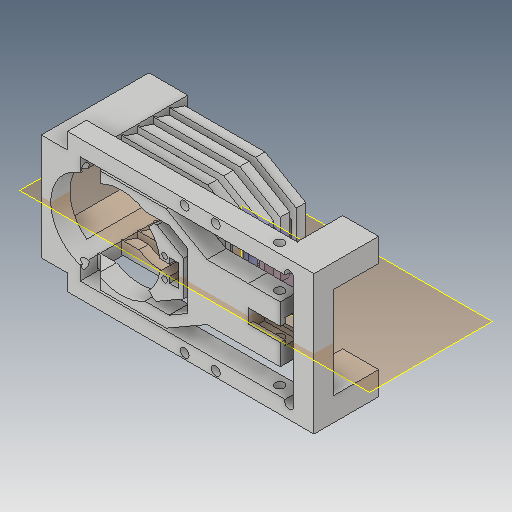
# Autodesk Inventor part: 20_focus_inlet_linearflexure_v1_1x1
Saved by Autodesk Inventor 2019.4 (Build 234330000, 330)
## iProperties
Created: 2020-02-03
Part Number: 20_focus_inlet_linearflexure_v1_1x1
Material: Generic
Document SubType Name: Modeling
Designer: diederichbenedict
Density: 1 g/cm^3
Appearance: Default
Author: diederichbenedict
Autodesk Inventor part; units mm, degrees
ref_plane "Work Plane1" through (0, 0, 0) normal (0, 0, 1) x (1, 0, 0)
sketch "Sketch1" plane through (0, 0, 0) normal (0, 0, 1) x (1, 0, 0)
  line L0 (33.5, -15.3849) -> (35.5, -15.3849) projected
  line L1 (35.5, -15.3849) -> (35.5, -14.1603) projected
  arc A0 (35.5, -14.1603) -> (35.3294, -13.8326) centre (35.1, -14.1603) ccw projected
  line L2 (35.3294, -13.8326) -> (34.0923, -12.9664) projected
  arc A1 (33.8775, -12.693) -> (34.0923, -12.9664) centre (34.4364, -12.4749) ccw projected
  arc A2 (33.8775, -12.693) -> (33.8775, -21.107) centre (23.1, -16.9) ccw projected
  arc A3 (34.0923, -20.8336) -> (33.8775, -21.107) centre (34.4364, -21.3251) ccw construction
  line L3 (34.0923, -20.8336) -> (35.3294, -19.9674) construction
  arc A4 (35.3294, -19.9674) -> (35.5, -19.6397) centre (35.1, -19.6397) ccw construction
  line L4 (35.5, -19.6397) -> (35.5, -18.4151) construction
  line L5 (35.5, -18.4151) -> (33.5, -18.4151) construction
  line L6 (33.5, -18.4151) -> (33.5, -15.3849) projected
  line L7 (30.0099, -20.9316) -> (30.0099, -25.4) construction
  line L8 (30.0099, -25.4) -> (27.6057, -25.4) construction
  line L9 (27.6057, -25.4) -> (27.6057, -23.5105) construction
  arc A5 (27.6057, -10.2895) -> (27.6057, -23.5105) centre (23.1, -16.9) ccw construction
  line L10 (27.6057, -10.2895) -> (27.6057, -8.4) construction
  line L11 (27.6057, -8.4) -> (30.0099, -8.4) construction
  line L12 (30.0099, -8.4) -> (30.0099, -12.8684) projected
  arc A6 (30.0099, -20.9316) -> (30.0099, -12.8684) centre (23.1, -16.9) ccw projected
  line L13 (23.1, -16.9) -> (97.1528, -16.9) construction
  line L14 (35.4811, -18.415) -> (35.4811, -19.6397) construction
  arc A7 (35.3186, -19.9519) -> (35.4811, -19.6397) centre (35.1, -19.6397) ccw construction
  line L15 (35.3186, -19.9519) -> (34.0815, -20.8182) construction
  arc A8 (34.0815, -20.8182) -> (33.8599, -21.1001) centre (34.4364, -21.3251) ccw construction
  line L16 (35.7169, -15.385) -> (35.7169, -16.9) construction
  line L17 (35.7169, -15.385) -> (35.7169, -16.9)
  line L18 (23.1, -16.9) -> (31.3304, -8.6696)
  line L19 (23.1, -16.9) -> (34.7396, -16.9) construction
  line L20 (31.3304, -8.6696) -> (33.4518, -6.5482)
  line L21 (33.4518, -6.5482) -> (34.3134, -6.5482)
  line L22 (42.7169, -11.4) -> (42.7169, -16.9)
  line L23 (35.7169, -16.9) -> (42.7169, -16.9)
  line L24 (35.7169, -16.9) -> (41.2169, -16.9)
  line L25 (41.2169, -16.9) -> (41.2169, -15.2)
  line L26 (41.2169, -15.2) -> (35.7169, -15.2)
  line L27 (35.7169, -15.2) -> (35.7169, -16.9)
  line L28 (41.2169, -15.2) -> (38.2169, -15.2)
  line L29 (38.2169, -15.2) -> (38.2169, -13.4)
  line L30 (38.2169, -13.4) -> (41.2169, -13.4)
  line L31 (41.2169, -13.4) -> (41.2169, -15.2)
  line L32 (33.4518, -6.5482) -> (34.3134, -6.5482) construction
  line L33 (42.7169, -11.4) -> (34.3134, -6.5482)
  line L34 (42.7169, -11.4) -> (52.4204, -11.4) construction
  arc A9 (31.3304, -8.6696) -> (30.0099, -7.5334) centre (23.1, -16.9) ccw construction
  arc A10 (28.2242, -6.5482) -> (33.8599, -21.1001) centre (23.1, -16.9) ccw construction
  arc A11 (33.8599, -21.1001) -> (33.9142, -20.9583) centre (23.1, -16.9) ccw
  arc A12 (34.6422, -15.3971) -> (31.3304, -8.6696) centre (23.1, -16.9) ccw
  line L35 (35.7169, -15.2) -> (34.6148, -15.2)
  circle A13 centre (36.7119, -13.6943) radius 0.9
  point P0 (0, 0)
  dimension "d1" = 45
  dimension "d2" = 3
  dimension "d6" = 1.7
  dimension "d8" = 3.5
  dimension "d9" = 3
  dimension "d147" = 7
  dimension "d148" = 120
  dimension "d149" = 5.5
  dimension "d155" = 12.6169
  dimension "d156" = 1.8
  dimension "d162" = 1.5
  constraints: 46 end point, 13 point on circle, 8 horizontal, 7 centre point, 6 point on line, 4 parallel, 4 perpendicular, 2 collinear, 2 equal length, 1 coincident, 3 other
  measures "d1" angle of L19 L18
  measures "d2" distance of L18.end L20.end
  measures "d6" distance of L25.end L24.end
  measures "d8" distance between parallel lines of L13 L30
  measures "d9" distance between parallel lines of L31 L29
  measures "d147" distance of L16.end L22.end
  measures "d148" angle of L22 L33
  measures "d149" distance of L22.start L22.end
  measures "d155" distance from line of L16 A2.centre
  measures "d156" diameter of A13
  measures "d162" distance between parallel lines of L31 L22
extrude "Extrusion1" add sketch "Sketch1" against normal blind 35 contours A12 A1 L2 A0 L1 L35 | L1 A0 L2 A1 A12 L20 L21 L33 L22 L23 L25 L31 L30 L29 L26 L35
sketch "Sketch2" plane through (0, 0, 0) normal (0, 0, 1) x (1, 0, 0)
  line L0 (41.2169, -13.4) -> (41.2169, -16.9) projected
  line L1 (42.7169, -16.9) -> (41.2169, -16.9) projected
  line L2 (42.7169, -11.4) -> (42.7169, -16.9) projected
  line L3 (31.3304, -8.6696) -> (33.4518, -6.5482) projected
  line L4 (34.6148, -15.2) -> (38.2169, -15.2) projected
  line L5 (38.2169, -15.2) -> (38.2169, -13.4) projected
  line L6 (38.2169, -13.4) -> (41.2169, -13.4) projected
  line L7 (95.8, 0) -> (0, 0) projected
  line L8 (6, -33.8) -> (89.8, -33.8) projected
  line L9 (6, -33.8) -> (6, 0) projected
  line L10 (11, -0.7) -> (45.4618, -0.7)
  line L11 (11, -4.7) -> (11, -0.7)
  line L12 (44.0169, -4.6174) -> (44.0169, -16.9)
  line L13 (44.0169, -16.9) -> (50.0084, -16.9)
  line L14 (50.0084, -16.9) -> (50.0084, -8.0766)
  line L15 (6.2, -0.1) -> (10.2, -0.1)
  line L16 (10.2, -0.1) -> (10.2, -16.9)
  line L17 (10.2, -16.9) -> (6.2, -16.9)
  line L18 (6.2, -16.9) -> (6.2, -0.1)
  line L19 (50.0084, -16.9) -> (63.0169, -16.9)
  line L20 (63.0169, -16.9) -> (63.0169, -8.0766)
  line L21 (63.0169, -8.0766) -> (50.0084, -8.0766)
  line L22 (50.0084, -8.0766) -> (50.0084, -16.9)
  arc A0 (79.6921, -19.4) -> (79.6921, -14.4) centre (79.6921, -16.9) ccw projected
  line L23 (58.0169, -7.7662) -> (58.0169, -8.0766)
  line L24 (6.2, -0.1) -> (10.2, -0.1)
  line L25 (10.2, -0.1) -> (10.2, 4.9)
  line L26 (10.2, 4.9) -> (6.2, 4.9)
  line L27 (6.2, 4.9) -> (6.2, -0.1)
  line L28 (1.6162, -33.8) -> (1.6162, 0) projected
  line L29 (-2, 0) -> (1.6162, 0) projected
  line L30 (-2, -33.8) -> (-2, 0) projected
  line L31 (1.6162, -33.8) -> (-2, -33.8) projected
  line L32 (6.2, -16.9) -> (-2, -16.9)
  line L33 (-2, -16.9) -> (-2, -0.2)
  line L34 (-2, -0.2) -> (6.2, -0.2)
  line L35 (6.2, -0.2) -> (6.2, -16.9)
  line L36 (-2, 0) -> (0, 0) projected
  line L37 (10.2, 4.9) -> (89.6, 4.9)
  line L38 (89.6, 4.9) -> (89.6, 0)
  line L39 (89.6, 0) -> (10.2, 0)
  line L40 (10.2, 0) -> (10.2, 4.9)
  line L41 (89.8, 0) -> (89.8, 4.5) projected
  line L42 (95.8, 0) -> (89.8, 0) projected
  line L43 (97.8, -41.8) -> (97.8, 0) construction
  line L44 (94.1838, 0) -> (94.1838, -33.8) projected
  line L45 (97.8, -33.8) -> (94.1838, -33.8) projected
  line L46 (97.8, -33.8) -> (97.8, 0) projected
  line L47 (94.1838, 0) -> (97.8, 0) projected
  line L48 (97.8, -0.2) -> (85.8, -0.2)
  line L49 (85.8, -0.2) -> (85.8, -4.2)
  line L50 (85.8, -4.2) -> (97.8, -4.2)
  line L51 (97.8, -4.2) -> (97.8, -0.2)
  line L52 (85.8, -0.2) -> (89.6, -0.2)
  line L53 (89.6, -0.2) -> (89.6, 0)
  line L54 (89.6, 0) -> (85.8, 0)
  line L55 (85.8, 0) -> (85.8, -0.2)
  line L56 (34.3134, -6.5482) -> (42.7169, -11.4) projected
  line L57 (33.4518, -6.5482) -> (34.3134, -6.5482) projected
  line L58 (44.0169, -8.0815) -> (38.1599, -4.7)
  line L59 (44.0169, -8.0815) -> (50.78, -8.0815) construction
  line L60 (37.2316, -0.7) -> (50.0084, -8.0766)
  line L61 (37.2316, -0.7) -> (51.9849, -0.7) construction
  line L62 (38.1599, -4.7) -> (11, -4.7)
  line L63 (97.8, -4.2) -> (94.1838, -4.2)
  line L64 (94.1838, -4.2) -> (94.1838, -16.9)
  line L65 (94.1838, -16.9) -> (97.8, -16.9)
  line L66 (97.8, -16.9) -> (97.8, -4.2)
  line L67 (63.0169, -8.0766) -> (58.0169, -8.0766)
  line L68 (58.0169, -8.0766) -> (58.0169, -9.9)
  line L69 (58.0169, -9.9) -> (63.0169, -9.9)
  line L70 (63.0169, -9.9) -> (63.0169, -8.0766)
  circle A1 centre (23.1, -16.9) radius 10 projected
  circle A2 centre (23.1, -16.9) radius 12.5 projected
  arc A3 (30.5513, -4.7) -> (15.6487, -4.7) centre (23.1, -16.9) ccw
  arc A4 (34.6148, -15.2) -> (31.3304, -8.6696) centre (23.1, -16.9) ccw projected
  dimension "d12" = 5
  dimension "d13" = 0.7
  dimension "d15" = 4
  dimension "d16" = 0.2
  dimension "d25" = 5
  dimension "d28" = 0.1
  dimension "d29" = 5
  dimension "d30" = 0.2
  dimension "d31" = 0.2
  dimension "d32" = 12
  dimension "d33" = 4
  dimension "d34" = 0.2
  dimension "d59" = 1.3
  dimension "d68" = 7
  dimension "d150" = 4
  dimension "d151" = 3
  constraints: 94 end point, 22 parallel, 12 horizontal, 11 point on line, 9 perpendicular, 2 equal length, 2 point on circle, 1 centre point, 1 coincident, 1 midpoint
  measures "d12" distance between parallel lines of L11 L9
  measures "d13" distance between parallel lines of L10 L7
  measures "d15" distance of L16.end L17.end
  measures "d16" distance between parallel lines of L18 L9
  measures "d25" distance between parallel lines of L20 L23
  measures "d28" distance between parallel lines of L7 L15
  measures "d29" distance of L25.end L24.end
  measures "d30" distance between parallel lines of L34 L36
  measures "d31" distance between parallel lines of L41 L38
  measures "d32" distance of L50.end L49.end
  measures "d33" distance of L49.end L48.end
  measures "d34" distance between parallel lines of L7 L48
  measures "d59" distance between parallel lines of L12 L2
  measures "d68" distance between parallel lines of L69 L19
  measures "d150" distance between parallel lines of L10 L62
  measures "d151" distance between parallel lines of L60 L58
extrude "Extrusion2" add sketch "Sketch2" against normal blind 6 contours L62 L11 L10 L60 L12 L58 A3 | L12 L60 L14 L13 | L21 L68 L69 L20 L19 L14 | L21 L20 L69 L68 | L48 L46 L50 L44 | L44 L50 L49 L48 | L53 L48 L55 L7 | L7 L25 L37 L38 | L50 L46 L65 L44 | L25 L15 L27 L7 | L7 L27 L26 L25 | L16 L17 L18 L15 | L34 L18 L32 L9 | L9 L32 L28 L34 | L28 L32 L30 L34
sketch "Sketch3" plane through (0, 0, -6) normal (0, 0, 1) x (1, 0, 0)
  line L0 (44.0169, -8.0815) -> (44.0169, -16.9) projected
  line L1 (44.0169, -16.9) -> (63.0169, -16.9) projected
  line L2 (63.0169, -8.0766) -> (63.0169, -16.9) projected
  line L3 (63.0169, -8.0766) -> (50.0084, -8.0766) projected
  line L4 (37.2316, -0.7) -> (11, -0.7) projected
  line L5 (11, -0.7) -> (11, -4.7) projected
  line L6 (41.2169, -13.4) -> (41.2169, -16.9) projected
  line L7 (42.7169, -16.9) -> (41.2169, -16.9) projected
  line L8 (42.7169, -11.4) -> (42.7169, -16.9) projected
  line L9 (31.3304, -8.6696) -> (33.4518, -6.5482) projected
  line L10 (34.6148, -15.2) -> (38.2169, -15.2) projected
  line L11 (38.2169, -15.2) -> (38.2169, -13.4) projected
  line L12 (38.2169, -13.4) -> (41.2169, -13.4) projected
  line L13 (6.2, 4.9) -> (6.2, -0.2) projected
  line L14 (-2, -16.9) -> (10.2, -16.9) projected
  line L15 (10.2, -16.9) -> (10.2, 0) projected
  line L16 (11, -4.7) -> (11, -0.7) projected
  line L17 (10.2, 0) -> (10.2, -16.9) projected
  line L18 (11, -0.7) -> (10.2, -0.7)
  line L19 (10.2, -0.7) -> (10.2, -4.7)
  line L20 (10.2, -4.7) -> (11, -4.7)
  line L21 (11, -4.7) -> (11, -0.7)
  line L22 (44.0169, -16.9) -> (44.0169, -8.0815) projected
  line L23 (42.7169, -16.9) -> (44.0169, -16.9)
  line L24 (44.0169, -16.9) -> (44.0169, -11.4)
  line L25 (44.0169, -11.4) -> (42.7169, -11.4)
  line L26 (42.7169, -11.4) -> (42.7169, -16.9)
  line L27 (6.2, -0.2) -> (-2, -0.2) projected
  line L28 (-2, -0.2) -> (-2, -16.9) projected
  line L29 (89.6, 4.9) -> (6.2, 4.9) projected
  line L30 (10.2, 0) -> (85.8, 0) projected
  line L31 (89.6, -0.2) -> (89.6, 4.9) projected
  line L32 (85.8, 0) -> (85.8, -4.2) projected
  line L33 (85.8, -4.2) -> (94.1838, -4.2) projected
  line L34 (97.8, -16.9) -> (97.8, -0.2) projected
  line L35 (97.8, -0.2) -> (89.6, -0.2) projected
  line L36 (33.4518, -6.5482) -> (34.3134, -6.5482) projected
  line L37 (50.0084, -8.0766) -> (37.2316, -0.7) projected
  line L38 (30.5513, -4.7) -> (38.1599, -4.7) projected
  line L39 (38.1599, -4.7) -> (44.0169, -8.0815) projected
  line L40 (94.1838, -4.2) -> (94.1838, -16.9) projected
  line L41 (94.1838, -16.9) -> (97.8, -16.9) projected
  line L42 (11, -4.7) -> (15.6487, -4.7) projected
  arc A0 (30.5513, -4.7) -> (15.6487, -4.7) centre (23.1, -16.9) ccw projected
  line L43 (34.3134, -6.5482) -> (42.7169, -11.4) projected
  arc A1 (34.6148, -15.2) -> (31.3304, -8.6696) centre (23.1, -16.9) ccw projected
  point P0 (0, 0)
  point P1 (42, -4.4)
  point P2 (10.2, -0.1)
  point P3 (10.2, 4.9)
  dimension "d152" = 0
  constraints: 16 end point, 4 parallel, 2 horizontal, 2 perpendicular, 1 point on line, 2 other
  measures "d152" distance from line of L8.start L25
extrude "Extrusion3" add sketch "Sketch3" along normal blind 0.5 contours L0 L23 L8 L25 | L20 L15 L18 L5
sketch "Sketch5" plane through (0, 0, -6) normal (0, 0, -1) x (-1, 0, 0)
  line L0 (2, -16.9) -> (2, -0.2) projected
  line L1 (2, -0.2) -> (-6.2, -0.2) projected
  line L2 (-6.2, -0.2) -> (-6.2, 4.9) projected
  line L3 (-6.2, 4.9) -> (-89.6, 4.9) projected
  line L4 (-89.6, 4.9) -> (-89.6, -0.2) projected
  line L5 (-89.6, -0.2) -> (-97.8, -0.2) projected
  line L6 (-97.8, -0.2) -> (-97.8, -16.9) projected
  line L7 (-94.1838, -4.2) -> (-85.8, -4.2) projected
  line L8 (-85.8, -4.2) -> (-85.8, 0) projected
  line L9 (-85.8, 0) -> (-10.2, 0) projected
  line L10 (-10.2, 0) -> (-10.2, -0.7) projected
  line L11 (-10.2, -16.9) -> (2, -16.9) projected
  line L12 (-97.8, -16.9) -> (-94.1838, -16.9) projected
  line L13 (-94.1838, -16.9) -> (-94.1838, -4.2) projected
  line L14 (-10.2, -4.7) -> (-10.2, -0.7) projected
  arc A0 (-1, -16.9) -> (-10.2, -4.3971) centre (-14.0958, -16.9) ccw
  line L15 (-10.2, -4.7) -> (-10.2, -16.9) projected
  line L16 (-37.2316, -0.7) -> (-10.2, -0.7) projected
  line L17 (-37.2316, -0.7) -> (-50.0084, -8.0766) projected
  line L18 (-50.0084, -8.0766) -> (-63.0169, -8.0766) projected
  line L19 (-63.0169, -8.0766) -> (-63.0169, -16.9) projected
  line L20 (-63.0169, -16.9) -> (-42.7169, -16.9) projected
  line L21 (-42.7169, -11.4) -> (-42.7169, -16.9) projected
  line L22 (-44.0169, -8.0815) -> (-38.1599, -4.7) projected
  line L23 (-38.1599, -4.7) -> (-30.5513, -4.7) projected
  arc A1 (-15.6487, -4.7) -> (-30.5513, -4.7) centre (-23.1, -16.9) ccw projected
  line L24 (-15.6487, -4.7) -> (-10.2, -4.7) projected
  line L25 (-44.0169, -11.4) -> (-42.7169, -11.4) projected
  line L26 (-44.0169, -11.4) -> (-44.0169, -8.0815) projected
  dimension "d65" = 0
  dimension "d66" = 3
  constraints: 2 point on circle, 1 centre point, 1 point on line
  measures "d65" distance from line of A0.centre L11
  measures "d66" distance from line of L0 A0.start
extrude "Extrusion5" cut sketch "Sketch5" against normal through all contours L11 L15 L14 A0
sketch "Sketch6" plane through (0, 0, -6) normal (0, 0, -1) x (-1, 0, 0)
  line L0 (-50.0084, -8.0766) -> (-63.0169, -8.0766) projected
  line L1 (-63.0169, -8.0766) -> (-63.0169, -16.9) projected
  line L2 (-1, -16.9) -> (2, -16.9) construction
  line L3 (-10.2, 0) -> (-10.2, -0.7) projected
  line L4 (2, -0.2) -> (2, -16.9) projected
  line L5 (2, -0.2) -> (-10.2, -0.2)
  line L6 (2, -4.4) -> (2, -0.2)
  line L7 (2, -4.4) -> (2, -0.2) construction
  line L8 (2, -0.2) -> (-10.2, -0.2) construction
  line L9 (-37.2316, -0.7) -> (-50.0084, -8.0766) projected
  line L10 (-44.0169, -8.0815) -> (-38.1599, -4.7) projected
  line L11 (2, -4.4) -> (-10.2, -4.4)
  line L12 (-10.2, -4.4) -> (-10.2, -0.2)
  line L13 (-10.2, -0.2) -> (2, -0.2)
  line L14 (2, -0.2) -> (2, -4.4)
  line L15 (-38.1599, -4.7) -> (-30.5513, -4.7) projected
  arc A0 (-15.6487, -4.7) -> (-30.5513, -4.7) centre (-23.1, -16.9) ccw projected
  line L16 (-37.2316, -0.7) -> (-10.2, -0.7) projected
  line L17 (-63.0169, -16.9) -> (-42.7169, -16.9) projected
  line L18 (-42.7169, -11.4) -> (-42.7169, -16.9) projected
  line L19 (-15.6487, -4.7) -> (-10.2, -4.7) projected
  line L20 (-1, -16.9) -> (2, -16.9) projected
  line L21 (-37.2316, -0.7) -> (-10.2, -0.7) projected
  line L22 (-37.2316, -0.7) -> (-50.0084, -8.0766) projected
  line L23 (-50.0084, -8.0766) -> (-63.0169, -8.0766) projected
  line L24 (-63.0169, -8.0766) -> (-63.0169, -16.9) projected
  line L25 (-63.0169, -16.9) -> (-42.7169, -16.9) projected
  line L26 (-42.7169, -11.4) -> (-42.7169, -16.9) projected
  line L27 (-44.0169, -8.0815) -> (-38.1599, -4.7) projected
  line L28 (-38.1599, -4.7) -> (-30.5513, -4.7) projected
  arc A1 (-15.6487, -4.7) -> (-30.5513, -4.7) centre (-23.1, -16.9) ccw projected
  line L29 (-15.6487, -4.7) -> (-10.2, -4.7) projected
  line L30 (-10.2, -4.7) -> (-10.2, -4.3971) projected
  arc A2 (-1, -16.9) -> (-10.2, -4.3971) centre (-14.0958, -16.9) ccw projected
  line L31 (-10.2, -4.7) -> (-10.2, -4.3971) projected
  arc A3 (-1, -16.9) -> (-10.2, -4.3971) centre (-14.0958, -16.9) ccw projected
  line L32 (2, -16.9) -> (2, -0.2) projected
  line L33 (2, -0.2) -> (-6.2, -0.2) projected
  line L34 (-6.2, -0.2) -> (-6.2, 4.9) projected
  line L35 (-6.2, 4.9) -> (-89.6, 4.9) projected
  line L36 (-89.6, 4.9) -> (-89.6, -0.2) projected
  line L37 (-89.6, -0.2) -> (-97.8, -0.2) projected
  line L38 (-97.8, -0.2) -> (-97.8, -16.9) projected
  line L39 (-97.8, -16.9) -> (-94.1838, -16.9) projected
  line L40 (-94.1838, -16.9) -> (-94.1838, -4.2) projected
  line L41 (-94.1838, -4.2) -> (-85.8, -4.2) projected
  line L42 (-85.8, -4.2) -> (-85.8, 0) projected
  line L43 (-85.8, 0) -> (-10.2, 0) projected
  line L44 (-10.2, 0) -> (-10.2, -0.7) projected
  line L45 (2, -16.9) -> (2, -0.2) projected
  line L46 (2, -0.2) -> (-6.2, -0.2) projected
  line L47 (-6.2, -0.2) -> (-6.2, 4.9) projected
  line L48 (-6.2, 4.9) -> (-89.6, 4.9) projected
  line L49 (-89.6, 4.9) -> (-89.6, -0.2) projected
  line L50 (-89.6, -0.2) -> (-97.8, -0.2) projected
  line L51 (-97.8, -0.2) -> (-97.8, -16.9) projected
  line L52 (-97.8, -16.9) -> (-94.1838, -16.9) projected
  line L53 (-94.1838, -16.9) -> (-94.1838, -4.2) projected
  line L54 (-94.1838, -4.2) -> (-85.8, -4.2) projected
  line L55 (-85.8, -4.2) -> (-85.8, 0) projected
  line L56 (-85.8, 0) -> (-10.2, 0) projected
  line L57 (-44.0169, -11.4) -> (-42.7169, -11.4) projected
  line L58 (-44.0169, -11.4) -> (-42.7169, -11.4) projected
  line L59 (-44.0169, -11.4) -> (-44.0169, -8.0815) projected
  line L60 (-44.0169, -11.4) -> (-44.0169, -8.0815) projected
  point P0 (0, 0)
  constraints: 16 end point, 2 horizontal, 2 parallel, 1 perpendicular
ref_plane "Work Plane2" through (6, 4.5, -33.8) normal (0, 0, 1) x (1, 0, 0)
extrude "Extrusion6" add sketch "Sketch6" along normal up to surface (27.8 mm away) contours L3 L5 L4 L11 A2 L12 | A2 L11 L12
ref_plane "Work Plane3" through (0, 0, -18) normal (0, 0, -1) x (-1, 0, 0)
sketch "Sketch7" plane through (0, 0, -18) normal (0, 0, -1) x (-1, 0, 0)
  line L0 (-11, -0.7) -> (-10.2, -0.7) projected
  line L1 (-10.2, -4.7) -> (-11, -4.7) projected
  line L2 (-11.9304, -0.7) -> (-11, -0.7) projected
  line L3 (-11.9304, -4.3971) -> (-11.9304, -0.7) projected
  line L4 (-50.0084, -8.0766) -> (-63.0169, -8.0766) projected
  line L5 (-63.0169, -8.0766) -> (-63.0169, -16.9) projected
  line L6 (-42.7169, -16.9) -> (-44.0169, -16.9) projected
  line L7 (-42.7169, -16.9) -> (-42.7169, -11.4) projected
  line L8 (-10.2, -0.2) -> (-10.2, -4.4) projected
  line L9 (2, -4.4) -> (2, -0.2) projected
  line L10 (2, -0.2) -> (-10.2, -0.2) projected
  line L11 (-37.2316, -0.7) -> (-50.0084, -8.0766) projected
  line L12 (-44.0169, -8.0815) -> (-38.1599, -4.7) projected
  line L13 (-11, -4.3971) -> (-11.9304, -4.3971) projected
  line L14 (-10.2, -4.4) -> (2, -4.4) projected
  line L15 (-38.1599, -4.7) -> (-30.5513, -4.7) projected
  arc A0 (-15.6487, -4.7) -> (-30.5513, -4.7) centre (-23.1, -16.9) ccw projected
  line L16 (-11, -0.7) -> (-11, -4.3971) projected
  line L17 (-44.0169, -11.4) -> (-44.0169, -16.9) projected
  line L18 (-37.2316, -0.7) -> (-10.2, -0.7) projected
  line L19 (-63.0169, -16.9) -> (-42.7169, -16.9) construction
  line L20 (-42.7169, -11.4) -> (-42.7169, -16.9) projected
  line L21 (-15.6487, -4.7) -> (-10.2, -4.7) projected
  line L22 (-11, -0.7) -> (-11, -4.7) projected
  line L23 (-10.2, -4.3971) -> (-10.2, -0.7) projected
  line L24 (-10.2, -4.4) -> (-10.2, -4.3971) projected
  line L25 (2, -4.4) -> (-10.1907, -4.4) projected
  line L26 (-1, -16.9) -> (2, -16.9) projected
  arc A1 (-1, -16.9) -> (-10.1907, -4.4) centre (-14.0958, -16.9) ccw projected
  line L27 (-10.2, -4.7) -> (-10.2, -4.3971) projected
  line L28 (-10.2, -4.3971) -> (-10.2, -0.7) projected
  line L29 (-10.2, -0.2) -> (-6.2, -0.2) projected
  line L30 (-6.2, -0.2) -> (-6.2, 4.9) projected
  line L31 (-6.2, 4.9) -> (-89.6, 4.9) projected
  line L32 (-89.6, 4.9) -> (-89.6, -0.2) projected
  line L33 (-89.6, -0.2) -> (-97.8, -0.2) projected
  line L34 (-97.8, -0.2) -> (-97.8, -16.9) projected
  line L35 (-97.8, -16.9) -> (-94.1838, -16.9) projected
  line L36 (-94.1838, -16.9) -> (-94.1838, -4.2) projected
  line L37 (-94.1838, -4.2) -> (-85.8, -4.2) projected
  line L38 (-85.8, -4.2) -> (-85.8, 0) projected
  line L39 (-85.8, 0) -> (-10.2, 0) projected
  line L40 (-10.2, 0) -> (-10.2, -0.2) projected
  line L41 (-10.2, -4.7) -> (-10.2, -4.4) projected
  line L42 (2, -16.9) -> (2, -4.4) projected
  line L43 (-44.0169, -11.4) -> (-42.7169, -11.4) projected
  line L44 (-44.0169, -11.4) -> (-42.7169, -11.4) projected
  line L45 (-63.0169, -8.0766) -> (-50.0084, -8.0766) projected
  line L46 (-50.0084, -8.0766) -> (-50.0084, -16.9)
  line L47 (-44.0169, -16.9) -> (-63.0169, -16.9) construction
  line L48 (-48.6166, -16.9) -> (-48.6166, -12.0219)
  line L49 (-50.0084, -16.9) -> (-48.6166, -16.9)
  line L50 (-37.2316, -0.7) -> (-50.0084, -8.0766) projected
  line L51 (-50.0084, -8.0766) -> (-37.2316, -0.7)
  line L52 (-37.2316, -0.7) -> (-10.2, -0.7) projected
  line L53 (-37.2316, -0.7) -> (-10.2, -0.7)
  line L54 (-10.2, -0.7) -> (-10.2, -4.7)
  line L55 (-44.0169, -12.0219) -> (-44.0169, -16.9) projected
  line L56 (-48.6166, -12.0219) -> (-38.1599, -4.7)
  line L57 (-38.1599, -4.7) -> (-30.5513, -4.7) projected
  line L58 (-38.1599, -4.7) -> (-30.5513, -4.7)
  line L59 (-15.6487, -4.7) -> (-10.2, -4.7) projected
  arc A2 (-15.6487, -4.7) -> (-30.5513, -4.7) centre (-23.1, -16.9) ccw
  line L60 (-44.0169, -11.4) -> (-44.0169, -8.0815) projected
  point P0 (0, 0)
  point P1 (-42, -16.9)
  point P2 (-58.0169, -11.1604)
  constraints: 16 end point, 4 collinear, 2 point on circle, 1 centre point, 1 parallel, 1 perpendicular, 1 point on line, 1 vertical, 2 other
extrude "Extrusion7" add sketch "Sketch7" along normal blind 3 contours L16 L13 L3 L2 | L0 L8 L27 L1 L22 L16 | L3 L13 L22 L21 A0 L15 L12 L60 L56 L48 L49 L46 L11 L18 | L56 L60 L12
sketch "Sketch8" plane through (0, 0, -18) normal (0, 0, 1) x (1, 0, 0)
  line L0 (11, -0.7) -> (10.2, -0.7) projected
  line L1 (10.2, -4.7) -> (11, -4.7) projected
  line L2 (42.7169, -16.9) -> (44.0169, -16.9) projected
  line L3 (42.7169, -16.9) -> (42.7169, -11.4) projected
  line L4 (44.0169, -11.4) -> (44.0169, -16.9) projected
  line L5 (11, -0.7) -> (11, -4.7) projected
  line L6 (10.2, -4.7) -> (10.2, -4.3971) projected
  line L7 (10.2, -4.3971) -> (10.2, -0.7) projected
  line L8 (44.0169, -11.4) -> (42.7169, -11.4) projected
  line L9 (48.6166, -16.9) -> (48.6166, -12.0219) projected
  line L10 (42.7169, -16.9) -> (44.4628, -16.9)
  line L11 (44.4628, -16.9) -> (44.4628, -11.4)
  line L12 (44.4628, -11.4) -> (42.7169, -11.4)
  line L13 (42.7169, -11.4) -> (42.7169, -16.9)
  point P0 (0, 0)
  point P1 (10.2, -4.4)
  constraints: 8 end point, 2 parallel, 1 horizontal, 1 perpendicular
extrude "Extrusion8" add sketch "Sketch8" against normal blind 0.5
sketch "Sketch9" plane through (10.2, -0.7, -18) normal (0, 1, 0) x (1, 0, 0)
  line L0 (0, -12) -> (0, 15.8) projected
  line L1 (0, 0.5) -> (0.755, 0.5)
  line L2 (0.755, 0.5) -> (1.9359, 3.0025)
  line L3 (1.9359, 3.0025) -> (0, 3.0025)
  line L4 (0, 0.5) -> (0, 3.0025)
  line L5 (27.0316, 0) -> (0, 0) projected
  point P0 (-10.2, -18)
  dimension "d153" = 0.5
  constraints: 8 end point, 2 point on line, 1 collinear, 1 horizontal, 1 parallel
  measures "d153" distance between parallel lines of L1 L5
extrude "Extrusion9" cut sketch "Sketch9" against normal up to surface (4 mm away)
sketch "Sketch10" plane through (0, 0, -6) normal (0, 0, -1) x (-1, 0, 0)
  arc A0 (-75.8, -1.5) -> (-75.8, 2.7) centre (-75.8, 0.6) ccw projected
  line L0 (-10.2, 0) -> (-10.2, -0.2) projected
  line L1 (-89.6, 4.9) -> (-72.3075, 4.9)
  line L2 (-72.3075, 4.9) -> (-72.3075, -2.4765)
  line L3 (-72.3075, -2.4765) -> (-89.6, -2.4765)
  line L4 (-89.6, -2.4765) -> (-89.6, 4.9)
  line L5 (-1, -16.9) -> (2, -16.9) projected
  line L6 (2, -4.4) -> (-10.1907, -4.4) projected
  arc A1 (-1, -16.9) -> (-10.1907, -4.4) centre (-14.0958, -16.9) ccw projected
  line L7 (-10.2, -4.4) -> (-10.2, -4.3971) projected
  line L8 (-37.2316, -0.7) -> (-10.2, -0.7) projected
  line L9 (-37.2316, -0.7) -> (-50.0084, -8.0766) projected
  line L10 (-50.0084, -8.0766) -> (-63.0169, -8.0766) projected
  line L11 (-63.0169, -8.0766) -> (-63.0169, -16.9) projected
  line L12 (-63.0169, -16.9) -> (-42.7169, -16.9) projected
  line L13 (-42.7169, -11.4) -> (-42.7169, -16.9) projected
  line L14 (-44.0169, -8.0815) -> (-38.1599, -4.7) projected
  line L15 (-38.1599, -4.7) -> (-30.5513, -4.7) projected
  arc A2 (-15.6487, -4.7) -> (-30.5513, -4.7) centre (-23.1, -16.9) ccw projected
  line L16 (-15.6487, -4.7) -> (-10.2, -4.7) projected
  line L17 (-10.2, -0.2) -> (-6.2, -0.2) projected
  line L18 (-6.2, -0.2) -> (-6.2, 4.9) projected
  line L19 (-6.2, 4.9) -> (-89.6, 4.9) projected
  line L20 (-89.6, 4.9) -> (-89.6, -0.2) projected
  line L21 (-89.6, -0.2) -> (-97.8, -0.2) projected
  line L22 (-97.8, -0.2) -> (-97.8, -16.9) projected
  line L23 (-97.8, -16.9) -> (-94.1838, -16.9) projected
  line L24 (-94.1838, -16.9) -> (-94.1838, -4.2) projected
  line L25 (-94.1838, -4.2) -> (-85.8, -4.2) projected
  line L26 (-85.8, -4.2) -> (-85.8, 0) projected
  line L27 (-85.8, 0) -> (-10.2, 0) projected
  line L28 (-10.2, -4.3971) -> (-10.2, -0.7) projected
  line L29 (-10.2, -4.7) -> (-10.2, -4.4) projected
  line L30 (2, -16.9) -> (2, -4.4) projected
  line L31 (-44.0169, -11.4) -> (-42.7169, -11.4) projected
  line L32 (-44.0169, -11.4) -> (-44.0169, -8.0815) projected
  point P0 (0, 0)
  constraints: 8 end point, 2 parallel, 1 horizontal, 1 perpendicular
ref_plane "Work Plane4" through (10.2, -4.4, -20.3) normal (0, 0, -1) x (-1, 0, 0)
extrude "Extrusion10" add sketch "Sketch10" along normal up to surface (14.3 mm away) contours L27 L26 L3 L4 L1 L2 | L2 L3 L26 L27
sketch "Sketch11" plane through (89.6, 4.9, -20.3) normal (0, 0, -1) x (-1, 0, 0)
  arc A0 (13.8, -6.4) -> (13.8, -2.2) centre (13.8, -4.3) ccw projected
  circle A1 centre (13.8, -4.3) radius 1.4
  point P0 (89.6, -4.9)
  dimension "d54" = 2.8
  constraints: 1 centre point, 1 coincident
  measures "d54" diameter of A1
extrude "Extrusion11" cut sketch "Sketch11" against normal through all
sketch "Sketch12" plane through (0, 0, 0) normal (0, 0, 1) x (1, 0, 0)
  line L0 (77.9366, 6) -> (77.9366, 5) projected
  line L1 (77.9366, 5) -> (67.8634, 5) projected
  line L2 (67.8634, 5) -> (67.8634, 6) projected
  line L3 (0, 6) -> (67.8634, 6) projected
  line L4 (0, 0) -> (0, 6) projected
  line L5 (95.8, 0) -> (0, 0) projected
  line L6 (95.8, 0) -> (95.8, 6) projected
  line L7 (77.9366, 6) -> (95.8, 6) projected
  circle A0 centre (43, 3.1) radius 1.4 projected
  circle A1 centre (92.8, 3.1) radius 1.4 projected
  circle A2 centre (3, 3.1) radius 1.4 projected
  circle A3 centre (52.8, 3.1) radius 1.4 projected
extrude "Extrusion12" cut sketch "Sketch12" against normal through all contours A0 | A3
sketch "Sketch13" plane through (63.0169, -16.9, 0) normal (1, 0, 0) x (0, 0, -1)
  line L0 (5.5, 5.5) -> (5.5, 0) construction
  line L1 (0, 0) -> (5.5, 0) projected
  line L2 (0, 8.8185) -> (0, 0) projected
  line L3 (0, 8.8185) -> (6, 8.8185) projected
  line L4 (6, 5.5) -> (6, 8.8185) projected
  line L5 (6, 5.5) -> (5.5, 5.5) construction
  line L6 (0, 0) -> (5.5, 0) projected
  line L7 (6, 0) -> (6, 2.2)
  line L8 (0, 2.2) -> (0, 0)
  line L9 (1.5, 2.2) -> (1.5, 3.8)
  line L10 (1.5, 3.8) -> (5, 3.8)
  line L11 (5, 3.8) -> (5, 2.2)
  line L12 (0, 0) -> (6, 0) projected
  line L13 (5.5, 0) -> (6, 0)
  line L14 (6, 0) -> (6, 8.8185)
  line L15 (6, 8.8185) -> (0, 8.8185)
  line L16 (0, 8.8185) -> (0, 0)
  line L17 (0, 2.2) -> (0, 0)
  line L18 (5.5, 0) -> (6, 0)
  line L19 (6, 0) -> (6, 2.2)
  line L20 (5, 2.2) -> (5, 3.8)
  line L21 (5, 3.8) -> (1.5, 3.8)
  line L22 (1.5, 3.8) -> (1.5, 2.2)
  line L23 (6, 2.2) -> (5, 2.2)
  line L24 (1.5, 2.2) -> (0, 2.2)
  line L25 (6, 2.2) -> (5, 2.2)
  line L26 (1.5, 2.2) -> (0, 2.2)
  line L27 (0, 0) -> (1.5, 0)
  line L28 (5, 0) -> (5.5, 0)
  line L29 (6, 2.2) -> (6, 8.8185)
  line L30 (6, 8.8185) -> (0, 8.8185)
  line L31 (0, 8.8185) -> (0, 2.2)
  line L32 (0, 8.2304) -> (0, 1.7) projected
  line L33 (0, 2.2) -> (1.5, 2.2)
  line L34 (1.5, 2.2) -> (1.5, 3.8)
  line L35 (1.5, 3.8) -> (5, 3.8)
  line L36 (5, 2.2) -> (5, 3.8)
  line L37 (5, 2.2) -> (6, 2.2)
  point P0 (0, 16.9)
  point P1 (0, 18.6)
  point P2 (0, 21.4)
  point P3 (0, 18.6)
  point P4 (0, 21.4)
  dimension "d166" = 2.2
  dimension "d167" = 1
  dimension "d168" = 3.5
  dimension "d169" = 3.8
  constraints: 58 end point, 12 parallel, 11 perpendicular, 5 horizontal, 3 point on line, 1 collinear, 1 vertical
  measures "d166" distance of L7.end L7.start
  measures "d167" distance between parallel lines of L11 L4
  measures "d168" distance between parallel lines of L11 L9
  measures "d169" distance between parallel lines of L1 L10
extrude "Extrusion13" add sketch "Sketch13" along normal blind 10 contours L2 L3 L4 L14 L23 L11 L10 L9 L24
mirror "Mirror1" about plane through (6.2, -16.9, 0) normal (0, -1, 0) of "Extrusion1", "Extrusion2", "Extrusion3", "Extrusion5", "Extrusion6", "Extrusion7", "Extrusion8", "Extrusion9", "Extrusion10", "Extrusion11", "Extrusion12", "Extrusion13"
sketch "Sketch14" plane through (58.0169, -8.0815, 0) normal (0, 1, 0) x (1, 0, 0)
  line L0 (9.3, 20.8) -> (9.3, 18.3)
  line L1 (31.5831, 0) -> (-51.8169, 0) projected
  line L2 (31.5831, 0) -> (31.5831, 20.3) projected
  line L3 (31.5831, 20.3) -> (14.2906, 20.3) projected
  line L4 (14.2906, 6) -> (14.2906, 20.3) projected
  line L5 (-51.8169, 6) -> (14.2906, 6) projected
  line L6 (-51.8169, 0) -> (-51.8169, 6) projected
  circle A0 centre (11.813, 3) radius 1.45
  point P0 (-58.0169, 0)
  point P1 (14.3156, 19.0518)
  dimension "d69" = 2.9
  constraints: 2 end point, 1 centre point, 1 vertical, 3 other
  measures "d69" diameter of A0
extrude "Extrusion14" cut sketch "Sketch14" along normal through all both and the other way through all contours A0
sketch "Sketch15" plane through (89.6, 4.9, -20.3) normal (0, 0, -1) x (-1, 0, 0)
  circle A0 centre (13.8, -4.3) radius 1.4 projected
  line L0 (0, 0) -> (17.2925, 0) projected
  line L1 (0, -7.3765) -> (0, 0) projected
  line L2 (17.2925, -7.3765) -> (0, -7.3765) projected
  line L3 (17.2925, 0) -> (17.2925, -7.3765) projected
  line L4 (-0.2, -38.7) -> (83.6, -38.7) projected
  circle A1 centre (13.8, -39.3) radius 1.4 projected
  line L5 (0, -43.6) -> (17.2925, -43.6) projected
  line L6 (17.2925, -43.6) -> (17.2925, -36.2235) projected
  line L7 (17.2925, -36.2235) -> (0, -36.2235) projected
  line L8 (0, -36.2235) -> (0, -43.6) projected
  line L9 (0, -36.2235) -> (3.8, -36.2235) projected
  line L10 (0, -43.6) -> (17.2925, -43.6) projected
  line L11 (0, -36.2235) -> (6, -36.2235)
  line L12 (6, -36.2235) -> (6, -43.6)
  line L13 (6, -43.6) -> (0, -43.6)
  line L14 (0, -43.6) -> (0, -36.2235)
  line L15 (0, 0) -> (17.2925, 0) projected
  line L16 (0, -7.3765) -> (6, -7.3765)
  line L17 (6, -7.3765) -> (6, 0)
  line L18 (6, 0) -> (0, 0)
  line L19 (0, 0) -> (0, -7.3765)
  point P0 (89.6, -4.9)
  dimension "d72" = 6
  constraints: 16 end point, 4 parallel, 3 point on line, 2 horizontal, 2 perpendicular
  measures "d72" distance of L12.end L13.end
extrude "Extrusion15" add sketch "Sketch15" along normal up to surface (13.5 mm away) contours L0 L17 L2 L1 | L8 L7 L12 L4 | L4 L12 L5 L8
sketch "Sketch16" plane through (0, 0, -6) normal (0, 0, -1) x (-1, 0, 0)
  line L0 (-10.1907, -29.4) -> (2, -29.4) construction
  line L1 (2, -4.4) -> (-10.1907, -4.4) construction
  line L2 (-10.1907, -4.4) -> (2, -4.4)
  line L3 (-10.1907, -29.4) -> (2, -29.4)
  line L4 (2, -29.4) -> (2, -27.4)
  line L5 (2, -33.6) -> (2, -33.6) projected
  line L6 (2, -27.4) -> (-6.2696, -27.4)
  arc A0 (-10.2, -29.4029) -> (-10.2, -4.3971) centre (-14.0958, -16.9) ccw projected
  line L7 (2, -4.4) -> (2, -6.4)
  line L8 (2, -6.4) -> (-6.2696, -6.4)
  arc A1 (-10.1907, -29.4) -> (-6.2696, -27.4) centre (-14.0958, -16.9) ccw
  arc A2 (-6.2696, -6.4) -> (-10.1907, -4.4) centre (-14.0958, -16.9) ccw
  line L9 (-10.2, 0) -> (-10.2, -0.2) projected
  line L10 (-10.2, -29.4029) -> (-10.2, -29.4) projected
  line L11 (-10.2, -29.1) -> (-15.6487, -29.1) projected
  arc A3 (-30.5513, -29.1) -> (-15.6487, -29.1) centre (-23.1, -16.9) ccw projected
  line L12 (-38.1599, -29.1) -> (-30.5513, -29.1) projected
  line L13 (-44.0169, -25.7185) -> (-38.1599, -29.1) projected
  line L14 (-42.7169, -11.4) -> (-42.7169, -22.4) projected
  line L15 (-44.0169, -8.0815) -> (-38.1599, -4.7) projected
  line L16 (-38.1599, -4.7) -> (-30.5513, -4.7) projected
  arc A4 (-15.6487, -4.7) -> (-30.5513, -4.7) centre (-23.1, -16.9) ccw projected
  line L17 (-15.6487, -4.7) -> (-10.2, -4.7) projected
  line L18 (-37.2316, -0.7) -> (-10.2, -0.7) projected
  line L19 (-37.2316, -0.7) -> (-50.0084, -8.0766) projected
  line L20 (-50.0084, -8.0766) -> (-63.0169, -8.0766) projected
  line L21 (-63.0169, -14.7) -> (-63.0169, -19.1) projected
  line L22 (-50.0084, -25.7234) -> (-63.0169, -25.7234) projected
  line L23 (-10.2, -33.1) -> (-37.2316, -33.1) projected
  line L24 (-10.2, -4.3971) -> (-10.2, -0.7) projected
  arc A5 (-10.1907, -29.4) -> (-10.1907, -4.4) centre (-14.0958, -16.9) ccw projected
  line L25 (-10.2, -4.4) -> (-10.2, -4.3971) projected
  line L26 (-72.3075, 4.9) -> (-72.3075, 0) projected
  line L27 (-72.3075, 0) -> (-10.2, 0) projected
  line L28 (-10.2, -0.2) -> (-6.2, -0.2) projected
  line L29 (-6.2, -0.2) -> (-6.2, 4.9) projected
  line L30 (-6.2, 4.9) -> (-72.3075, 4.9) projected
  line L31 (-72.3075, -33.8) -> (-72.3075, -38.7) projected
  line L32 (-6.2, -38.7) -> (-72.3075, -38.7) projected
  line L33 (-6.2, -33.6) -> (-6.2, -38.7) projected
  line L34 (-6.2, -33.6) -> (-10.2, -33.6) projected
  line L35 (-10.2, -33.8) -> (-10.2, -33.6) projected
  line L36 (-72.3075, -33.8) -> (-10.2, -33.8) projected
  line L37 (2, -4.4) -> (2, -29.4) projected
  line L38 (-10.2, -33.1) -> (-10.2, -29.4029) projected
  line L39 (-10.2, -4.7) -> (-10.2, -4.4) projected
  line L40 (-44.0169, -11.4) -> (-42.7169, -11.4) projected
  line L41 (-37.2316, -33.1) -> (-50.0084, -25.7234) projected
  line L42 (-44.0169, -22.4) -> (-42.7169, -22.4) projected
  line L43 (-10.2, -29.4) -> (-10.2, -29.1) projected
  line L44 (-44.0169, -22.4) -> (-44.0169, -25.7185) projected
  line L45 (-44.0169, -11.4) -> (-44.0169, -8.0815) projected
  line L46 (-63.0169, -8.0766) -> (-63.0169, -8.0815) projected
  line L47 (-63.0169, -8.0815) -> (-73.0169, -8.0815) projected
  line L48 (-73.0169, -14.7) -> (-73.0169, -8.0815) projected
  line L49 (-63.0169, -14.7) -> (-73.0169, -14.7) projected
  line L50 (-63.0169, -19.1) -> (-73.0169, -19.1) projected
  line L51 (-73.0169, -19.1) -> (-73.0169, -25.7185) projected
  line L52 (-63.0169, -25.7185) -> (-73.0169, -25.7185) projected
  line L53 (-63.0169, -25.7185) -> (-63.0169, -25.7234) projected
  point P0 (0, 0)
  point P1 (2, -0.2)
  dimension "d76" = 2
  dimension "d77" = 2
  constraints: 12 end point, 5 point on circle, 2 centre point, 2 concentric, 2 perpendicular, 2 other
  measures "d76" distance of L3.end L4.end
  measures "d77" distance of L2.end L7.end
extrude "Extrusion16" add sketch "Sketch16" along normal up to surface (27.8 mm away) contours L2 L7 L8 A0 | L6 L4 L3 A0
sketch "Sketch17" plane through (-2, -0.2, -33.8) normal (-1, 0, 0) x (0, 0, 1)
  line L0 (33.8, 0) -> (0, 0) construction
  line L1 (0, -6.2) -> (0, 0) construction
  line L2 (27.8, -6.2) -> (0, -6.2) construction
  line L3 (27.8, -6.2) -> (27.8, -27.2) construction
  line L4 (27.8, -27.2) -> (0, -27.2) construction
  line L5 (0, -27.2) -> (0, -33.4) construction
  line L6 (33.8, -33.4) -> (0, -33.4) construction
  line L7 (32.15, -3.5) -> (1.65, -3.5) construction
  line L8 (1.65, -3.5) -> (1.65, -29.9) construction
  line L9 (1.65, -29.9) -> (32.15, -29.9) construction
  line L10 (32.15, -29.9) -> (32.15, -3.5) construction
  line L11 (32.15, -3.5) -> (1.65, -29.9) construction
  line L12 (1.65, -3.5) -> (32.15, -29.9) construction
  circle A0 centre (1.65, -29.9) radius 1.5 construction
  circle A1 centre (1.65, -3.5) radius 1.5 construction
  circle A2 centre (32.15, -3.5) radius 1.5 construction
  circle A3 centre (32.15, -29.9) radius 1.5 construction
  circle A4 centre (1.65, -29.9) radius 1.2
  circle A5 centre (1.65, -3.5) radius 1.2
  circle A6 centre (32.15, -29.9) radius 1.2
  circle A7 centre (32.15, -3.5) radius 1.2
  line L13 (33.8, 0) -> (33.8, -33.4) projected
  point P0 (33.8, 0.2)
  point P1 (16.9, -16.7)
  dimension "d80" = 30.5
  dimension "d81" = 26.4
  dimension "d82" = 3
  dimension "d83" = 3
  dimension "d84" = 3
  dimension "d85" = 3
  dimension "d89" = 0.3
  dimension "d90" = 0.3
  dimension "d91" = 0.3
  dimension "d92" = 0.3
  constraints: 12 end point, 8 centre point, 4 coincident, 2 midpoint, 2 parallel, 1 horizontal, 1 perpendicular
  measures "d80" distance of L9.end L8.end
  measures "d81" distance of L8.end L7.end
  measures "d82" diameter of A0
  measures "d83" diameter of A1
  measures "d84" diameter of A2
  measures "d85" diameter of A3
  measures "d89" radial gap between concentric circles of A0 A4
  measures "d90" radial gap between concentric circles of A1 A5
  measures "d91" radial gap between concentric circles of A3 A6
  measures "d92" radial gap between concentric circles of A2 A7
extrude "Extrusion17" cut sketch "Sketch17" against normal up to surface (12.2 mm away)
ref_plane "Work Plane8" through (72.3075, -16.9, -6) normal (0, 1, 0) x (1, 0, 0)
ref_plane "Work Plane9" through (61, -9.9, -11) normal (0, 0, -1) x (-1, 0, 0)
sketch "Sketch23" plane through (61, -9.9, -11) normal (0, 0, -1) x (-1, 0, 0)
  line L0 (18.2831, -1.5) -> (18.2831, -12.5) projected
  line L1 (18.2831, -12.5) -> (16.5372, -12.5) projected
  line L2 (18.2831, -1.5) -> (16.5372, -1.5) projected
  line L3 (16.5372, -1.5) -> (16.5372, -12.5) projected
  point P0 (61, 9.9)
extrude "Extrusion23" cut sketch "Sketch23" against normal blind 8
sketch "Sketch24" plane through (0, 0, -6) normal (0, 0, 1) x (1, 0, 0)
  line L0 (42.7169, -11.4) -> (42.7169, -22.4) projected
  line L1 (42.7169, -22.4) -> (44.4628, -22.4) projected
  line L2 (42.7169, -11.4) -> (44.4628, -11.4) projected
  line L3 (44.4628, -11.4) -> (44.4628, -22.4) projected
  point P0 (0, 0)
extrude "Extrusion24" add sketch "Sketch24" along normal up to surface (0.5 mm away)
chamfer "Chamfer2" distance 5.5 angle 45 2 edges at (11, -2.7, 0) (11, -31.1, 0)
sketch "Sketch25" plane through (89.6, -31.3235, -33.8) normal (0, 0, -1) x (-1, 0, 0)
  line L0 (6, 0) -> (0, 0) construction
  line L1 (0, 0) -> (0, -7.3765) construction
  line L2 (0, -7.3765) -> (6, -7.3765) construction
  line L3 (6, -7.3765) -> (6, 0) construction
  line L4 (0, 36.2235) -> (0, 28.8471) construction
  line L5 (0, 28.8471) -> (6, 28.8471) construction
  line L6 (6, 28.8471) -> (6, 36.2235) construction
  line L7 (6, 36.2235) -> (0, 36.2235) construction
  line L8 (0, 0) -> (3.8, 0) construction
  line L9 (3.8, 1.7235) -> (3.8, 0) construction
  line L10 (-4.5838, 1.7235) -> (3.8, 1.7235) construction
  line L11 (-4.5838, 27.1235) -> (-4.5838, 1.7235) construction
  line L12 (-4.5838, 27.1235) -> (3.8, 27.1235) construction
  line L13 (3.8, 27.1235) -> (3.8, 28.8471) construction
  line L14 (3.8, 28.8471) -> (0, 28.8471) construction
  line L15 (0, 28.8471) -> (0, 31.1235) construction
  line L16 (0, 31.1235) -> (-8.2, 31.1235) construction
  line L17 (-8.2, 31.1235) -> (-8.2, -2.2765) construction
  line L18 (0, -2.2765) -> (-8.2, -2.2765) construction
  line L19 (0, -2.2765) -> (0, 0) construction
  line L20 (6, 0) -> (6, -7.3765) projected
  line L21 (6, -7.3765) -> (-8.2, -7.3765)
  line L22 (-8.2, -7.3765) -> (-8.2, 36.2235)
  line L23 (-8.2, 36.2235) -> (6, 36.2235)
  line L24 (6, 36.2235) -> (6, -7.3765)
  point P0 (89.6, 31.3235)
  constraints: 8 end point, 2 parallel, 1 horizontal, 1 perpendicular
extrude "Extrusion25" cut sketch "Sketch25" against normal through all
sketch "Sketch26" plane through (77.0649, -33.8, 0) normal (0, 1, 0) x (1, 0, 0)
  line L0 (6.5351, 0) -> (6.5351, 6) projected
  line L1 (6.5351, 6) -> (0, 6) projected
  line L2 (0, 6) -> (0, 0) projected
  line L3 (0, 0) -> (6.5351, 0) projected
  point P0 (-77.0649, 0)
extrude "Extrusion26" add sketch "Sketch26" along normal up to next
pattern_linear "Rectangular Pattern1" count 3 spacing 5 along (0, 0, -1) count 2 spacing 5 along (0, 0, 1) of "Extrusion7", "Extrusion8", "Extrusion9"
mirror "Mirror3" about plane through (72.3075, -16.9, -6) normal (0, 1, 0) of "Extrusion7", "Extrusion8", "Extrusion9", "Rectangular Pattern1"
sketch "Sketch29" plane through (0, 0, -35) normal (0, 0, -1) x (-1, 0, 0)
  circle A0 centre (-36.7119, -20.1057) radius 0.9 projected
  circle A1 centre (-36.7119, -13.6943) radius 0.9 projected
  line L0 (-41.2169, -20.4) -> (-41.2169, -13.4) projected
  line L1 (-41.2169, -13.4) -> (-38.2169, -13.4) projected
  line L2 (-38.2169, -13.4) -> (-38.2169, -15.2) projected
  line L3 (-38.2169, -15.2) -> (-34.6148, -15.2) projected
  arc A2 (-31.3304, -8.6696) -> (-34.6148, -15.2) centre (-23.1, -16.9) ccw projected
  line L4 (-31.3304, -8.6696) -> (-33.4518, -6.5482) projected
  line L5 (-33.4518, -6.5482) -> (-34.3134, -6.5482) projected
  line L6 (-34.3134, -6.5482) -> (-42.7169, -11.4) projected
  line L7 (-42.7169, -11.4) -> (-42.7169, -22.4) projected
  line L8 (-34.3134, -27.2518) -> (-42.7169, -22.4) projected
  line L9 (-33.4518, -27.2518) -> (-34.3134, -27.2518) projected
  line L10 (-31.3304, -25.1304) -> (-33.4518, -27.2518) projected
  arc A3 (-34.6148, -18.6) -> (-31.3304, -25.1304) centre (-23.1, -16.9) ccw projected
  line L11 (-38.2169, -18.6) -> (-34.6148, -18.6) projected
  line L12 (-38.2169, -20.4) -> (-38.2169, -18.6) projected
  line L13 (-41.2169, -20.4) -> (-38.2169, -20.4) projected
  circle A4 centre (-23.1, -16.9) radius 12.25
  point P0 (0, 0)
  dimension "d157" = 24.5
  constraints: 1 centre point, 1 coincident
  measures "d157" diameter of A4
extrude "Extrusion29" cut sketch "Sketch29" against normal up to surface (35 mm away) contours A4 L3 A2 L4 L10 A3 L11 | L11 A3 L10 A4 | A4 L4 A2 L3
ref_plane "Work Plane5" through (6, -38.3, -33.8) normal (0, 0, -1) x (1, 0, 0)
ref_plane "Work Plane6" through (10.2, -29.4, -20.3) normal (0, 0, 1) x (-1, 0, 0)
ref_plane "Work Plane7" through (0, -33.8, -18) normal (0, 0, 1) x (-1, 0, 0)
body "Solid1"
